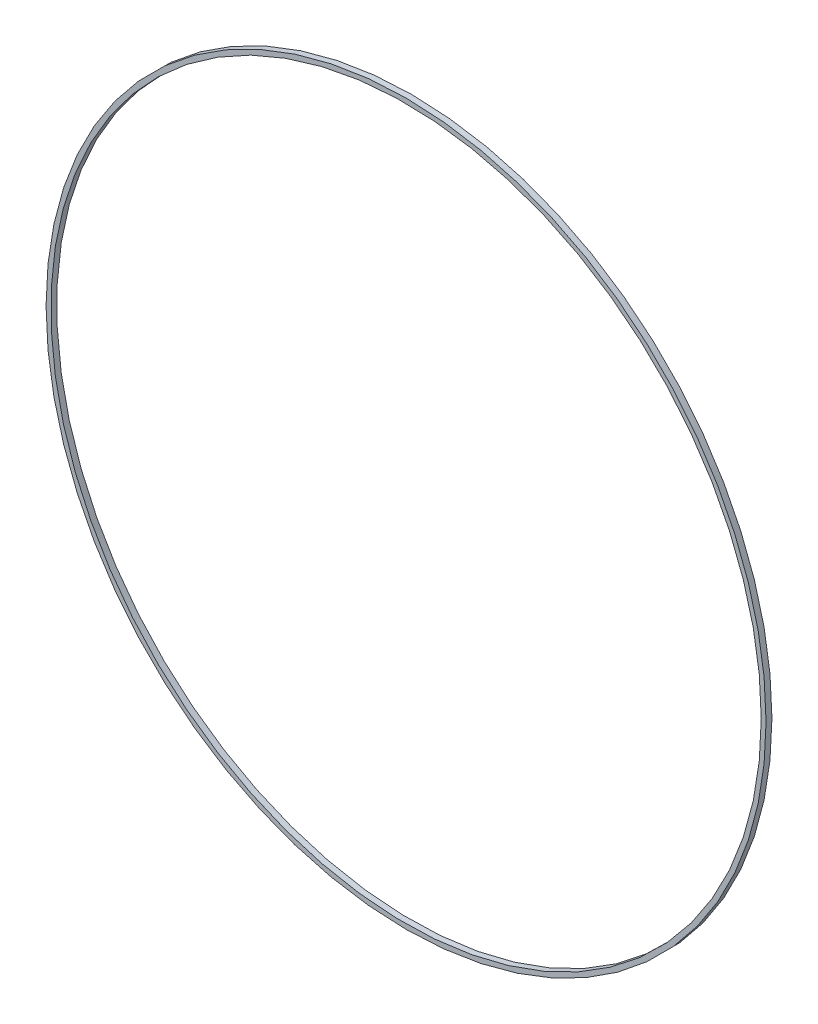
# Autodesk Inventor part: 零件3
Saved by Autodesk Inventor 2020 (Build 240168000, 168)
## iProperties
Created: 2021-06-27
Part Number: 零件3
Material: 常规
Document SubType Name: Modeling
Designer: chenpeizhi66
Density: 1 g/cm^3
Appearance: 默认
Author: chenpeizhi66
Autodesk Inventor part; units mm, degrees
ref_plane "YZ Plane" through (0, 0, 0) normal (1, 0, 0) x (0, 1, 0)
ref_plane "XZ Plane" through (0, 0, 0) normal (0, 1, 0) x (-1, 0, 0)
ref_plane "XY Plane" through (0, 0, 0) normal (0, 0, 1) x (1, 0, 0)
sketch "草图1" plane through (0, 0, 0) normal (0, 0, 1) x (1, 0, 0)
  circle A0 centre (0, 0) radius 75 projected
  circle A1 centre (0, 0) radius 74 projected
  point P0 (0, 0)
ref_plane "工作平面1" through (-136.6024, -136.6024, -1.225) normal (0, 0, 1) x (0.8660267, -0.4999977, 0)
extrude "拉伸1" add sketch "草图1" against normal up to surface (1.225 mm away)
